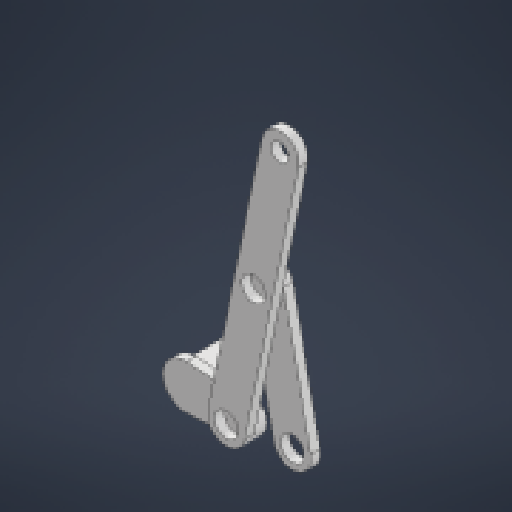
# Autodesk Inventor part: FrontLinkage
Saved by Autodesk Inventor 2024.1 (Build 281209000, 209)
## iProperties
Created: 2023-11-14
Part Number: FrontLinkage
Material: Generic
Document SubType Name: Modeling
Designer: Brandon
Density: 1 g/cm^3
Appearance: Default
Author: Brandon
Autodesk Inventor part; units mm, degrees
ref_plane "YZ Plane" through (0, 0, 0) normal (1, 0, 0) x (0, 1, 0)
ref_plane "XZ Plane" through (0, 0, 0) normal (0, 1, 0) x (-1, 0, 0)
ref_plane "XY Plane" through (0, 0, 0) normal (0, 0, 1) x (1, 0, 0)
sketch "Sketch1" plane through (0, 0, 0) normal (0, 0, 1) x (1, 0, 0)
  line L0 (2.032, -2.032) -> (-2.032, -2.032) projected
  line L1 (2.032, 2.032) -> (2.032, -2.032) projected
  line L2 (-2.032, 2.032) -> (2.032, 2.032) projected
  line L3 (-2.032, -2.032) -> (-2.032, 2.032) projected
  circle A0 centre (0, 0) radius 3.81 projected
  circle A1 centre (9.144, 0) radius 3.175
  circle A2 centre (18.288, 0) radius 3.175
  circle A3 centre (13.716, 22.3981) radius 3.175
  line L4 (0.2646, 3.8008) -> (9.3645, 3.1673)
  line L5 (0.2646, -3.8008) -> (9.3645, -3.1673)
  line L6 (21.3989, 0.635) -> (16.8269, 23.0331)
  line L7 (15.1771, -0.635) -> (10.6051, 21.7631)
  circle A4 centre (18.288, 0) radius 2.032
  line L8 (1.9812, 1.9812) -> (1.9812, -1.9812)
  line L9 (1.9812, -1.9812) -> (-1.9812, -1.9812)
  line L10 (-1.9812, -1.9812) -> (-1.9812, 1.9812)
  line L11 (-1.9812, 1.9812) -> (1.9812, 1.9812)
  dimension "d0" = 6.35
  dimension "d1" = 6.35
  dimension "d2" = 6.35
  dimension "d3" = 4.064
  dimension "d6" = 0.0508
  constraints: 16 end point, 8 point on circle, 8 tangent, 4 centre point, 4 coincident, 5 other
  measures "d0" diameter of A1
  measures "d1" diameter of A2
  measures "d2" diameter of A3
  measures "d3" diameter of A4
  measures "d6" distance between parallel lines of L2 L11
extrude "Extrusion1" add sketch "Sketch1" along normal blind 1.5875 contours L0 L3 L2 L1 | A0 | A0 L4 A1 L5 | A1 | A2 | A2 L7 A3 L6 | A3 | L8 L9 L10 L11
extrude "Extrusion2" add sketch "Sketch1" against normal blind 7.0358 contours L8 L9 L10 L11
chamfer "Chamfer1" distance 0.127 angle 45 4 edges at (-1.9812, 0, -7.0358) (0, -1.9812, -7.0358) (1.9812, 0, -7.0358) (0, 1.9812, -7.0358)
sketch "Sketch2" plane through (0, 0, 1.5875) normal (0, 0, 1) x (1, 0, 0)
  line L0 (0.2646, -3.8008) -> (9.3645, -3.1673) projected
  arc A0 (9.3645, -3.1673) -> (9.3645, 3.1673) centre (9.144, 0) ccw projected
  line L1 (9.3645, 3.1673) -> (0.2646, 3.8008) projected
  arc A1 (0.2646, 3.8008) -> (0.2646, -3.8008) centre (0, 0) ccw projected
  line L2 (21.3989, 0.635) -> (16.8269, 23.0331) projected
  arc A2 (16.8269, 23.0331) -> (10.6051, 21.7631) centre (13.716, 22.3981) ccw projected
  line L3 (10.6051, 21.7631) -> (15.1771, -0.635) projected
  arc A3 (15.1771, -0.635) -> (21.3989, 0.635) centre (18.288, 0) ccw projected
  circle A4 centre (18.288, 0) radius 2.032 projected
  circle A5 centre (9.144, 0) radius 3.175
  circle A6 centre (13.716, 22.3981) radius 3.175
  point P0 (10.6051, 21.7631)
  constraints: 2 coincident, 1 centre point, 1 concentric, 3 other
extrude "Extrusion3" add sketch "Sketch2" along normal blind 0.508 contours A5 A0 | A6 A2
sketch "Sketch3" plane through (9.144, 0, 2.0955) normal (0, 0, 1) x (1, 0, 0)
  circle A0 centre (0, 0) radius 3.175 projected
  circle A1 centre (4.572, 22.3981) radius 3.175 projected
  circle A2 centre (4.572, 22.3981) radius 1.905
  circle A3 centre (0, 0) radius 1.905
  circle A4 centre (0, 0) radius 2.032
  circle A5 centre (4.572, 22.3981) radius 2.032
  line L0 (1.4611, 21.7631) -> (6.0331, -0.635) projected
  line L1 (3.1109, -0.635) -> (7.6829, 21.7631)
  circle A6 centre (4.572, 22.3981) radius 3.175 projected
  line L2 (-3.1109, 0.635) -> (1.4611, 23.0331)
  circle A7 centre (0, 0) radius 3.175 projected
  arc A8 (12.2549, 44.1613) -> (6.0331, 45.4313) centre (9.144, 44.7963) ccw
  line L3 (1.4611, 23.0331) -> (6.0331, 45.4313)
  line L4 (7.6829, 21.7631) -> (12.2549, 44.1613)
  circle A9 centre (9.144, 44.7963) radius 1.524
  point P0 (-9.144, 0)
  point P1 (9.144, 36.576)
  point P2 (1.4611, 23.0331)
  point P3 (1.4611, 23.0331)
  dimension "d14" = 3.81
  dimension "d15" = 3.81
  dimension "d16" = 0.127
  dimension "d17" = 0.127
  dimension "d18" = 6.35
  dimension "d20" = 3.048
  constraints: 9 end point, 7 point on circle, 7 tangent, 6 centre point, 4 coincident, 2 other
  measures "d14" diameter of A2
  measures "d15" diameter of A3
  measures "d16" radial gap between concentric circles of A3 A4
  measures "d17" radial gap between concentric circles of A2 A5
  measures "d18" diameter of A8
  measures "d20" diameter of A9
extrude "Extrusion4" add sketch "Sketch3" along normal blind 1.5875 contours A0 | A0 L2 A1 L0 L1 | L3 A8 L4 A1 | A1 | L0 A1 L1
extrude "Extrusion5" cut sketch "Sketch3" along normal blind 0.2032 contours A0 | A0 L2 A1 L0 L1 | A1 | L0 A1 L1 | A4 | A5
extrude "Extrusion6" add sketch "Sketch3" along normal blind 2.3813 contours A2 | A3
sketch "Sketch4" plane through (9.144, 0, 4.4768) normal (0, 0, 1) x (1, 0, 0)
  circle A0 centre (4.572, 22.3981) radius 1.905 projected
  circle A1 centre (0, 0) radius 1.905 projected
  circle A2 centre (4.572, 22.3981) radius 1.905 projected
  circle A3 centre (4.572, 22.3981) radius 3.175
  circle A4 centre (0, 0) radius 2.032 projected
  circle A5 centre (0, 0) radius 3.175
  point P0 (-9.144, 0)
  dimension "d27" = 6.35
  dimension "d28" = 6.35
  constraints: 2 centre point, 2 coincident
  measures "d27" diameter of A3
  measures "d28" diameter of A5
extrude "Extrusion7" add sketch "Sketch4" against normal blind 0.5906 contours A0 | A1 | A3 | A4 | A5
sketch "Sketch5" plane through (0, 0, 1.5875) normal (0, 0, 1) x (1, 0, 0)
  circle A0 centre (0, 0) radius 1.524
  dimension "d31" = 3.048
  constraints: 1 centre point, 1 coincident
  measures "d31" diameter of A0
extrude "Extrusion8" cut sketch "Sketch5" against normal through all
chamfer "Chamfer2" distance 0.127 angle 45 2 edges at (-1.524, 0, 1.5875) (16.256, 0, 1.5875)
body "Solid1"
